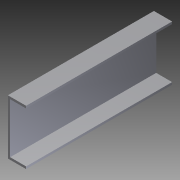
# Autodesk Inventor part: 1 by 3 U
Saved by Autodesk Inventor 2012 (Build 160160000, 160)
## iProperties
Created: 2013-09-05
Part Number: 1 by 3 U
Material: Default
Document SubType Name: Modeling
Designer: Bryce
Density: 1 g/cm^3
Author: Bryce
Autodesk Inventor part; units mm, degrees
ref_plane "YZ Plane" through (0, 0, 0) normal (1, 0, 0) x (0, 1, 0)
ref_plane "XZ Plane" through (0, 0, 0) normal (0, 1, 0) x (-1, 0, 0)
ref_plane "XY Plane" through (0, 0, 0) normal (0, 0, 1) x (1, 0, 0)
sketch "Sketch1" plane through (0, 0, 0) normal (0, 0, 1) x (1, 0, 0)
  line L0 (0, 0) -> (25.4, 0)
  line L1 (25.4, 76.2) -> (0, 76.2)
  line L2 (0, 76.2) -> (0, 0)
  line L3 (25.4, 73.025) -> (3.175, 73.025)
  line L4 (3.175, 73.025) -> (3.175, 3.175)
  line L5 (3.175, 3.175) -> (25.4, 3.175)
  line L6 (25.4, 0) -> (25.4, 3.175)
  line L7 (25.4, 73.025) -> (25.4, 76.2)
  dimension "d0" = 76.2
  dimension "d1" = 25.4
  dimension "d2" = 3.175
  dimension "d3" = 3.175
  dimension "d4" = 3.175
  constraints: 16 end point, 4 parallel, 3 perpendicular, 2 horizontal, 1 collinear
  measures "d0" distance of L1.end L0.start
  measures "d1" distance of L0.start L0.end
  measures "d2" distance between parallel lines of L1 L3
  measures "d3" distance between parallel lines of L2 L4
  measures "d4" distance between parallel lines of L0 L5
extrude "Extrusion1" add sketch "Sketch1" along normal blind 203.2
equation "\"d2\" = d3"
equation "\"d3\" = d4"
body "Solid1"
